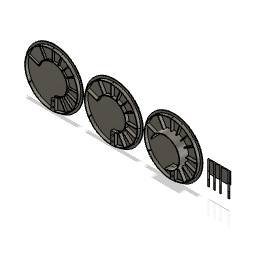
tray2 (Autodesk Fusion 360 design; units mm, degrees)
Autodesk Fusion 360 part; units mm, degrees
sketch "Sketch1" plane through (0, 0, 0) normal (0, 0, 1) x (1, 0, 0)
  circle A0 centre (0, 0) radius 48
  dimension "d1" = 96
  constraint coincident A0.centre origin
  measures "d1" diameter of A0
extrude "Extrude1" add sketch "Sketch1" along normal blind 1 makes body 1
sketch "Sketch2" plane through (0, 0, 1) normal (0, 0, 1) x (1, 0, 0)
  circle A0 centre (0, 0) radius 48
  circle A1 centre (0, 0) radius 44.5
  circle A2 centre (0, 0) radius 24
  line L0 (-21.3923, -12.4423) -> (-37.6324, -21.8186)
  line L1 (-0.3829, -44.4984) -> (-0.2151, -24.9991) construction
  line L2 (0.3829, -44.4984) -> (0.2151, -24.9991) construction
  line L3 (0.5, -43.4971) -> (0.5, -24.9949)
  line L4 (0.3829, -44.4984) -> (0.2151, -24.9991) construction
  line L5 (-0.3829, -44.4984) -> (-0.2151, -24.9991) construction
  line L6 (-0.5, -24.9949) -> (-0.5, -43.4971)
  line L7 (-0.5, -24.9949) -> (-0.5, -43.4971)
  line L8 (0.5, -43.4971) -> (0.5, -24.9949)
  line L9 (18.3655, -16.7159) -> (32.6713, -28.7199)
  line L10 (34.0108, -28.697) -> (18.8273, -16.1775) construction
  line L11 (24.4949, -1) -> (43.4885, -1)
  line L12 (24.4949, -1) -> (43.4885, -1)
  line L13 (33.3229, -27.9613) -> (19.012, -15.953)
  line L14 (33.5176, -29.2715) -> (18.5567, -16.4968) construction
  line L15 (21.1881, 11.801) -> (38.6377, 22.0767) construction
  line L16 (24.9983, -0.2892) -> (24.4991, -0.2935) construction
  line L17 (21.3911, 11.4445) -> (39.0085, 21.4147) construction
  line L18 (37.7117, 21.6814) -> (21.6901, 12.4313)
  line L19 (22.1701, 11.5537) -> (38.2001, 20.8087)
  line L20 (0.5, 23.9949) -> (0.5, 43.4971)
  line L21 (0.5, 23.9949) -> (0.5, 43.4971)
  line L22 (-0.2065, 23.9991) -> (-0.3829, 44.4984) construction
  line L23 (-0.5, 43.4971) -> (-0.5, 23.9949)
  line L24 (-0.5, 43.4971) -> (-0.5, 23.9949)
  line L25 (-0.2065, 23.9991) -> (-0.3829, 44.4984) construction
  line L26 (0.2065, 23.9991) -> (0.3829, 44.4984) construction
  line L27 (0.2065, 23.9991) -> (0.3829, 44.4984) construction
  line L28 (-41.1989, 13.9606) -> (-23.807, 7.6305)
  line L29 (-23.0959, 7.6749) -> (-42.1029, 14.4082) construction
  line L30 (-23.4828, 8.5767) -> (-40.8671, 14.904)
  line L31 (-22.9488, 8.0791) -> (-41.8448, 15.1414) construction
  line L32 (24.9899, -0.7107) -> (24.4991, -0.7065) construction
  line L33 (40.8861, -14.8517) -> (23.5018, -8.5243)
  line L34 (22.8458, -9.3498) -> (40.5339, -15.7877)
  line L35 (43.5, 0) -> (24.4949, 0)
  line L36 (43.5, 0) -> (24.4949, 0)
  line L37 (15.6609, 18.3411) -> (28.8963, 33.8416) construction
  line L38 (16.4495, 18.8259) -> (28.3424, 32.9993)
  line L39 (27.5764, 33.6421) -> (15.6835, 19.4687)
  line L40 (15.3395, 18.6037) -> (28.3097, 34.3338) construction
  line L41 (8.1841, 22.5927) -> (15.0198, 41.8886) construction
  line L42 (14.5672, 40.9884) -> (8.2395, 23.6032)
  line L43 (8.5722, 22.4514) -> (15.7379, 41.6241) construction
  line L44 (9.1769, 23.2548) -> (15.5056, 40.6427)
  line L45 (-12.1471, 21.8506) -> (-21.3978, 37.8733)
  line L46 (-11.9265, 20.9011) -> (-21.9916, 38.6861) construction
  line L47 (-12.3026, 20.6872) -> (-22.6701, 38.2925) construction
  line L48 (-22.2628, 37.3714) -> (-13.0112, 21.3473)
  line L49 (-37.1209, -22.6779) -> (-20.8871, -13.3054)
  line L50 (-38.0463, -23.0809) -> (-21.034, -13.0627) construction
  line L51 (-38.4413, -22.4168) -> (-21.2527, -12.6891) construction
  line L52 (21.8435, -38.77) -> (12.207, -21.7424) construction
  line L53 (11.9505, -21.8877) -> (21.2332, -37.9658)
  line L54 (22.1003, -37.4677) -> (12.8134, -21.3822)
  line L55 (22.4913, -38.3978) -> (12.5611, -21.5349) construction
  line L56 (44.4913, -0.8785) -> (43.4913, -0.8699) construction
  line L57 (24.9899, -0.7107) -> (24.4991, -0.7065) construction
  line L58 (44.4998, -0.1214) -> (43.4998, -0.13) construction
  line L59 (24.9983, -0.2892) -> (24.4991, -0.2935) construction
  line L60 (23.4011, -8.797) -> (23.0915, -8.6873) construction
  line L61 (41.5183, -16.0151) -> (40.5815, -15.665) construction
  line L62 (23.2505, -9.1877) -> (22.9502, -9.0754) construction
  arc A3 (40.8861, -14.8517) -> (43.4913, -0.8699) centre (0, 0) ccw
  arc A4 (19.1511, -16.0697) -> (23.2505, -9.1877) centre (0, 0) ccw
  arc A5 (12.8496, -21.445) -> (18.493, -16.8229) centre (0, 0) ccw
  arc A6 (33.2392, -28.0607) -> (40.5815, -15.665) centre (0, 0) ccw
  arc A7 (21.9839, -37.5361) -> (32.7571, -28.6221) centre (0, 0) ccw
  arc A8 (0.5, -24.995) -> (11.9817, -21.9417) centre (0, 0) ccw
  arc A9 (0.3743, -43.4984) -> (21.3509, -37.8997) centre (0, 0) ccw
  arc A10 (-37.1845, -22.5734) -> (-0.3743, -43.4984) centre (0, 0) ccw
  arc A11 (-21.0908, -13.423) -> (-0.5, -24.995) centre (0, 0) ccw
  arc A12 (-23.7203, 7.8961) -> (-21.6109, -12.5686) centre (0, 0) ccw
  arc A13 (-41.1602, 14.0743) -> (-37.571, -21.9242) centre (0, 0) ccw
  arc A14 (-12.7751, 21.4895) -> (-23.5771, 8.3139) centre (0, 0) ccw
  arc A15 (-22.1626, 37.4308) -> (-40.908, 14.7913) centre (0, 0) ccw
  arc A16 (-0.3743, 43.4984) -> (-21.4991, 37.8158) centre (0, 0) ccw
  arc A17 (14.6859, 40.946) -> (0.3743, 43.4984) centre (0, 0) ccw
  arc A18 (27.6735, 33.5623) -> (15.3878, 40.6874) centre (0, 0) ccw
  arc A19 (8.5082, 23.5077) -> (-12.3873, 21.7153) centre (0, 0) ccw
  arc A20 (15.9043, 19.2887) -> (8.911, 23.358) centre (0, 0) ccw
  arc A21 (21.8321, 12.1803) -> (16.2339, 19.0121) centre (0, 0) ccw
  arc A22 (43.4998, -0.13) -> (38.1381, 20.9221) centre (0, 0) ccw
  arc A23 (37.7759, 21.5692) -> (28.2469, 33.0811) centre (0, 0) ccw
  arc A24 (23.4011, -8.797) -> (24.98, -1) centre (0, 0) ccw
  arc A25 (24.9983, -0.2892) -> (22.0352, 11.8089) centre (0, 0) ccw
  dimension "d4" = 89
  dimension "d5" = 87
  dimension "d6" = 50
  dimension "d7" = 48
  constraint concentric A0 A1
  constraint concentric A0 A22
  constraint concentric A22 A24
  constraint concentric A1 A2
  constraint collinear L0 L18
  constraint collinear L6 L23
  constraint collinear L7 L24
  constraint collinear L28 L34
  constraint coincident A1 L61.start
  constraint coincident A1 L56.start
  constraint coincident A1 L58.start
  constraint coincident A1 L17.end
  constraint coincident A1 L15.end
  constraint coincident A1 L37.end
  constraint coincident A1 L40.end
  constraint coincident A1 L41.end
  constraint coincident A1 L43.end
  constraint coincident A1 L26.end
  constraint coincident A1 L22.end
  constraint coincident A1 L46.end
  constraint coincident A1 L47.end
  constraint coincident A1 L31.end
  constraint coincident A1 L29.end
  constraint coincident A1 L50.start
  constraint coincident A1 L51.start
  constraint coincident A1 L1.start
  constraint coincident A1 L2.start
  constraint coincident A1 L52.start
  constraint coincident A1 L55.start
  constraint coincident A1 L10.start
  constraint coincident A1 L14.start
  constraint coincident L11.end A22
  constraint coincident L35.start A22
  constraint collinear L56 L57
  constraint coincident L16.start A24
  constraint collinear L58 L59
  constraint collinear L61 L62
  constraint coincident L33.start A22
  constraint concentric A3 A22
  constraint coincident L34.end A22
  constraint coincident L33.end A24
  constraint concentric A4 A24
  constraint coincident L13 A4.start
  constraint coincident L9 A5.end
  constraint concentric A5 A24
  constraint coincident L54 A5.start
  constraint coincident L53 A8.end
  constraint coincident L14 A7.end
  constraint coincident L10 A6.start
  constraint concentric A6 A22
  constraint coincident A6 L13.start
  constraint coincident L9.end A22
  constraint coincident L54.start A22
  constraint coincident L53.end A22
  constraint coincident L52 A9.end
  constraint coincident L55 A7.start
  constraint concentric A7 A22
  constraint concentric A8 A24
  constraint coincident L3 A8.start
  constraint coincident L6 A11.end
  constraint coincident L1 A10.end
  constraint coincident L2 A9.start
  constraint concentric A9 A22
  constraint coincident A9 L3.start
  constraint coincident L6.end A22
  constraint coincident L49.start A22
  constraint coincident L0.end A22
  constraint coincident L51 A13.end
  constraint coincident L50 A10.start
  constraint concentric A10 A22
  constraint concentric A11 A24
  constraint coincident L49 A11.start
  constraint coincident L0 A12.end
  constraint coincident L28.end A24
  constraint coincident L30.start A24
  constraint coincident L31 A14.end
  constraint coincident L29 A12.start
  constraint concentric A12 A24
  constraint coincident L31 A15.end
  constraint coincident L29 A13.start
  constraint concentric A13 A22
  constraint coincident A13 L28.start
  constraint coincident L30.end A22
  constraint coincident L46 A19.end
  constraint coincident L47 A14.start
  constraint concentric A14 A24
  constraint coincident A14 L48.end
  constraint coincident L45.start A24
  constraint coincident L46 A16.end
  constraint coincident L47 A15.start
  constraint concentric A15 A22
  constraint coincident L45.end A22
  constraint coincident A15 L48.start
  constraint coincident L26 A17.end
  constraint coincident L22 A16.start
  constraint concentric A16 A22
  constraint coincident L20.end A22
  constraint coincident A16 L23.start
  constraint coincident L44.end A22
  constraint coincident L43 A18.end
  constraint coincident L41 A17.start
  constraint concentric A17 A22
  constraint coincident A17 L42.start
  constraint coincident L37 A23.end
  constraint coincident L40 A18.start
  constraint concentric A18 A22
  constraint coincident L38.end A22
  constraint coincident A18 L39.start
  constraint coincident L43 A20.end
  constraint coincident L41 A19.start
  constraint concentric A19 A24
  constraint coincident L44.start A24
  constraint coincident A19 L42.end
  constraint coincident L39.end A24
  constraint coincident L38.start A24
  constraint coincident L37 A21.end
  constraint coincident L40 A20.start
  constraint concentric A20 A24
  constraint coincident L19.start A24
  constraint coincident L18.end A24
  constraint coincident L17 A25.end
  constraint coincident L15 A21.start
  constraint concentric A21 A24
  constraint coincident L17 A22.end
  constraint coincident L15 A23.start
  constraint concentric A22 A23
  constraint coincident A22 L19.end
  constraint coincident A23 L18.start
  constraint concentric A24 A25
  constraint coincident L11 A24.end
  measures "d4" diameter of A1
  measures "d5" diameter of A22
  measures "d6" diameter of A24
  measures "d7" diameter of A2
extrude "Extrude3" add sketch "Sketch2" along normal blind 5 contours A1 | A2 L20 L21 L23 L24 A19 bodies 1
sketch "Sketch4" plane through (0, 0, 6) normal (0, 0, 1) x (1, 0, 0)
  arc A0 (27.5764, 33.6421) -> (15.5056, 40.6427) centre (0, 0) ccw
  line L0 (27.5764, 33.6421) -> (15.6835, 19.4687)
  arc A1 (15.6835, 19.4687) -> (9.1769, 23.2548) centre (0, 0) ccw
  line L1 (9.1769, 23.2548) -> (15.5056, 40.6427)
  arc A2 (40.8861, -14.8517) -> (43.4885, -1) centre (0, 0) ccw
  line L2 (40.8861, -14.8517) -> (23.5018, -8.5243)
  arc A3 (23.5018, -8.5243) -> (24.98, -1) centre (0, 0) ccw
  line L3 (24.98, -1) -> (43.4885, -1)
  arc A4 (-37.1209, -22.6779) -> (-0.5, -43.4971) centre (0, 0) ccw
  line L4 (-37.1209, -22.6779) -> (-21.0908, -13.423)
  arc A5 (-21.0908, -13.423) -> (-0.5, -24.995) centre (0, 0) ccw
  line L5 (-0.5, -24.995) -> (-0.5, -43.4971)
  arc A6 (0.5, -43.4971) -> (21.2332, -37.9658) centre (0, 0) ccw
  line L6 (0.5, -43.4971) -> (0.5, -24.995)
  arc A7 (0.5, -24.995) -> (11.9817, -21.9417) centre (0, 0) ccw
  line L7 (11.9817, -21.9417) -> (21.2332, -37.9658)
  arc A8 (33.3229, -27.9613) -> (40.5339, -15.7877) centre (0, 0) ccw
  line L8 (33.3229, -27.9613) -> (19.1511, -16.0697)
  arc A9 (19.1511, -16.0697) -> (23.142, -9.4576) centre (0, 0) ccw
  line L9 (23.142, -9.4576) -> (40.5339, -15.7877)
  arc A10 (-0.5, 43.4971) -> (-21.3978, 37.8733) centre (0, 0) ccw
  line L10 (-0.5, 43.4971) -> (-0.5, 24.995)
  arc A11 (-0.5, 24.995) -> (-12.1471, 21.8506) centre (0, 0) ccw
  line L11 (-12.1471, 21.8506) -> (-21.3978, 37.8733)
  arc A12 (14.5672, 40.9884) -> (0.5, 43.4971) centre (0, 0) ccw
  line L12 (14.5672, 40.9884) -> (8.2395, 23.6032)
  arc A13 (8.2395, 23.6032) -> (0.5, 24.995) centre (0, 0) ccw
  line L13 (0.5, 24.995) -> (0.5, 43.4971)
  arc A14 (22.1003, -37.4677) -> (32.6713, -28.7199) centre (0, 0) ccw
  line L14 (22.1003, -37.4677) -> (12.8496, -21.445)
  arc A15 (12.8496, -21.445) -> (18.493, -16.8229) centre (0, 0) ccw
  line L15 (18.493, -16.8229) -> (32.6713, -28.7199)
  arc A16 (37.7117, 21.6814) -> (28.3424, 32.9993) centre (0, 0) ccw
  line L16 (37.7117, 21.6814) -> (21.6901, 12.4313)
  arc A17 (21.6901, 12.4313) -> (16.4495, 18.8259) centre (0, 0) ccw
  line L17 (16.4495, 18.8259) -> (28.3424, 32.9993)
  arc A18 (-22.2628, 37.3714) -> (-40.8671, 14.904) centre (0, 0) ccw
  line L18 (-22.2628, 37.3714) -> (-13.0112, 21.3473)
  arc A19 (-13.0112, 21.3473) -> (-23.4828, 8.5767) centre (0, 0) ccw
  line L19 (-23.4828, 8.5767) -> (-40.8671, 14.904)
  arc A20 (-41.1989, 13.9606) -> (-37.6324, -21.8186) centre (0, 0) ccw
  line L20 (-41.1989, 13.9606) -> (-23.807, 7.6305)
  arc A21 (-23.807, 7.6305) -> (-21.6109, -12.5686) centre (0, 0) ccw
  line L21 (-21.6109, -12.5686) -> (-37.6324, -21.8186)
  arc A22 (43.5, 0) -> (38.2001, 20.8087) centre (0, 0) ccw
  line L22 (43.5, 0) -> (25, 0)
  arc A23 (25, 0) -> (22.1701, 11.5537) centre (0, 0) ccw
  line L23 (22.1701, 11.5537) -> (38.2001, 20.8087)
  circle A24 centre (0, 0) radius 24
  circle A25 centre (0, 0) radius 44.5
  circle A26 centre (0, 0) radius 24
  circle A27 centre (0, 0) radius 25
  constraint concentric A0 A26
  constraint concentric A26 A27
extrude "Extrude4" add sketch "Sketch4" along normal blind 10 contours A1 A3 A5 A7 A9 A11 A13 A15 A17 A19 A21 A23 A27 bodies 1
sketch "Sketch5" plane through (0, 0, 16) normal (0, 0, 1) x (1, 0, 0)
  circle A0 centre (0, 0) radius 24
  circle A1 centre (0, 0) radius 25
  line L0 (-0.5283, -25.9639) -> (-0.7943, 6.8859)
  line L1 (-0.7943, 6.8859) -> (-28.5016, 7.6395)
  line L2 (-28.5016, 7.6395) -> (-37.5896, -21.7967)
  line L3 (-37.5896, -21.7967) -> (-36.969, -22.7277)
  line L4 (-36.969, -22.7277) -> (-0.5283, -25.9639)
extrude "Extrude5" cut sketch "Sketch5" against normal up to surface (15 mm away) contours A0 L0 L1 | A0 A1 L0 L1 | A1 L0 L1 L2 L3 L4 picked at (-1.7694, -13.5925) picked at (-23.4288, 6.3815) bodies 1
sketch "Sketch6" plane through (0, 0, 0) normal (0, 1, 0) x (1, 0, 0)
  line L0 (90, 0) -> (115, -25)
  line L1 (115, -25) -> (116.4142, -23.5858)
  line L2 (92.2226, 0.6058) -> (92.2217, 0.6055)
  line L3 (101, -25) -> (102.4142, -23.5858)
  line L4 (78.2226, 0.6058) -> (78.2217, 0.6055)
  line L5 (76, 0) -> (101, -25)
  line L6 (91, -25) -> (92.4142, -23.5858)
  line L7 (68.2226, 0.6058) -> (68.2217, 0.6055)
  line L8 (66, 0) -> (91, -25)
  line L9 (81, -25) -> (82.4142, -23.5858)
  line L10 (58.2226, 0.6058) -> (58.2217, 0.6055)
  line L11 (56, 0) -> (81, -25)
  line L12 (56, -0.04) -> (56, 0)
  line L13 (92.8684, 0) -> (92.8684, -0.04)
  line L14 (92.8684, -0.04) -> (92.8684, 0.6055)
  line L15 (92.8684, 0.6055) -> (56, 0.6055)
  line L16 (56, 0.6055) -> (56, -0.04)
  line L17 (92.8284, 0) -> (92.8684, 0)
  line L18 (78.8284, 0) -> (90, 0)
  line L19 (102.4142, -23.5858) -> (78.8284, 0)
  line L20 (78.2229, 0.6055) -> (78.2226, 0.6058)
  line L21 (116.4142, -23.5858) -> (92.8284, 0)
  line L22 (92.2229, 0.6055) -> (92.2226, 0.6058)
  line L23 (58.8284, 0) -> (66, 0)
  line L24 (68.8284, 0) -> (76, 0)
  line L25 (56.04, -0.04) -> (56, -0.04)
  line L26 (92.4142, -23.5858) -> (68.8284, 0)
  line L27 (68.2229, 0.6055) -> (68.2226, 0.6058)
  line L28 (56, -0.04) -> (56.04, -0.04)
  line L29 (82.4142, -23.5858) -> (58.8284, 0)
  line L30 (58.2229, 0.6055) -> (58.2226, 0.6058)
  dimension "d29" = 2
  dimension "d30" = 2
  dimension "d31" = 2
  dimension "d32" = 2
  constraint perpendicular L0 L1
  constraint perpendicular L1 L21
  constraint perpendicular L3 L5
  constraint perpendicular L3 L19
  constraint perpendicular L6 L8
  constraint perpendicular L6 L26
  constraint perpendicular L9 L11
  constraint perpendicular L9 L29
  constraint vertical L12
  constraint horizontal L23
  constraint vertical L13
  constraint coincident L13.end L21
  constraint horizontal L28
  constraint vertical L14
  constraint horizontal L15
  constraint vertical L16
  constraint coincident L15 L2.end
  constraint collinear L17 L23
  constraint collinear L18 L23
  constraint coincident L15 L4.end
  constraint coincident L15 L20.start
  constraint collinear L19 L20
  constraint coincident L15 L22.start
  constraint collinear L21 L22
  constraint collinear L23 L24
  constraint coincident L15 L27.start
  constraint collinear L26 L27
  constraint coincident L15 L7.end
  constraint coincident L11 L25.start
  constraint coincident L15 L10.end
  constraint coincident L15 L30.start
  constraint collinear L29 L30
  measures "d29" distance of L0.end L1.end
  measures "d30" distance of L3.end L3.start
  measures "d31" distance of L6.end L6.start
  measures "d32" distance of L9.end L9.start
extrude "Extrude6" add sketch "Sketch6" along normal mid plane 20 separate body contours L0 L1 L3 L5 L6 L8 L9 L11 L14 L15 L16 L17 L18 L19 L21 L23 L24 L26 L29 makes body 2
sketch "Sketch7" plane through (56, 0, 0) normal (-1, 0, 0) x (0, 0, 1)
  line L0 (0, -10) -> (0, 10)
  line L1 (0, 10) -> (-0.6055, 10)
  line L2 (-0.6055, 10) -> (-0.6055, -10)
  line L3 (-0.6055, -10) -> (0, -10)
  line L4 (0, 20) -> (25, 5)
  line L5 (25, 5) -> (25, -5)
  line L6 (25, -5) -> (0, -15)
  line L7 (0, -15) -> (34.4485, -15)
  line L8 (34.4485, -15) -> (34.7895, 20.635)
  line L9 (34.7895, 20.635) -> (0, 20)
  constraint vertical L5
  constraint perpendicular L5 L7
extrude "Extrude7" cut sketch "Sketch7" against normal blind 78 contours L4 L5 L6 L7 L8 L9 bodies 2
extrude "Extrude8" add 1 faces at (80.579, 3.3333, -0.6055) along direction (0, 0, -1) blind 1 on bodies 2 bodies 2
copy_body "CopyPasteBodies1" bodies 1 makes body 3
move_body "Move1" bodies 3 to x (1, 0, 0) y (0, 1, 0) z (0, 0, 1) at (-100, 0, 0)
sketch "Sketch8" plane through (0, 0, 16) normal (0, 0, 1) x (1, 0, 0)
  line L0 (-100.5443, -23.9938) -> (-100.5362, -24.9943)
  arc A0 (-100.5362, -24.9943) -> (-123.8444, 7.5129) centre (-100, 0) ccw
  line L1 (-123.8444, 7.5129) -> (-122.8031, 7.4845)
  arc A1 (-100.5443, -23.9938) -> (-122.8031, 7.4845) centre (-100, 0) ccw
extrude "Extrude9" cut sketch "Sketch8" against normal up to surface (10 mm away) bodies 3
copy_body "CopyPasteBodies2" bodies 1 makes body 4
move_body "Move2" bodies 4 to x (1, 0, 0) y (0, 1, 0) z (0, 0, 1) at (-200, 0, 0)
sketch "Sketch9" plane through (0, 0, 6) normal (0, 0, 1) x (1, 0, 0)
  line L0 (-237.0351, -22.6284) -> (-237.5896, -21.7967)
  line L1 (-237.5896, -21.7967) -> (-237.5885, -21.7932)
  line L2 (-237.5885, -21.7932) -> (-237.6324, -21.8186)
  arc A0 (-241.1989, 13.9606) -> (-237.6324, -21.8186) centre (-200, 0) ccw
  line L3 (-241.1989, 13.9606) -> (-223.807, 7.6305)
  arc A1 (-223.4828, 8.5767) -> (-223.807, 7.6305) centre (-200, 0) ccw
  line L4 (-223.4828, 8.5767) -> (-240.8671, 14.904)
  arc A2 (-222.2628, 37.3714) -> (-240.8671, 14.904) centre (-200, 0) ccw
  line L5 (-222.2628, 37.3714) -> (-213.0112, 21.3473)
  arc A3 (-212.1471, 21.8506) -> (-213.0112, 21.3473) centre (-200, 0) ccw
  line L6 (-212.1471, 21.8506) -> (-221.3978, 37.8733)
  arc A4 (-200.5, 43.4971) -> (-221.3978, 37.8733) centre (-200, 0) ccw
  line L7 (-200.5, 43.4971) -> (-200.5, 24.995)
  arc A5 (-199.5, 24.995) -> (-200.5, 24.995) centre (-200, 0) ccw
  line L8 (-199.5, 24.995) -> (-199.5, 43.4971)
  arc A6 (-185.4328, 40.9884) -> (-199.5, 43.4971) centre (-200, 0) ccw
  line L9 (-185.4328, 40.9884) -> (-191.7605, 23.6032)
  arc A7 (-190.8231, 23.2548) -> (-191.7605, 23.6032) centre (-200, 0) ccw
  line L10 (-190.8231, 23.2548) -> (-184.4944, 40.6427)
  arc A8 (-172.4236, 33.6421) -> (-184.4944, 40.6427) centre (-200, 0) ccw
  line L11 (-172.4236, 33.6421) -> (-184.3165, 19.4687)
  arc A9 (-183.5505, 18.8259) -> (-184.3165, 19.4687) centre (-200, 0) ccw
  line L12 (-183.5505, 18.8259) -> (-171.6576, 32.9993)
  arc A10 (-162.2883, 21.6814) -> (-171.6576, 32.9993) centre (-200, 0) ccw
  line L13 (-162.2883, 21.6814) -> (-178.3099, 12.4313)
  arc A11 (-177.8299, 11.5537) -> (-178.3099, 12.4313) centre (-200, 0) ccw
  line L14 (-177.8299, 11.5537) -> (-161.7999, 20.8087)
  arc A12 (-156.5, 0) -> (-161.7999, 20.8087) centre (-200, 0) ccw
  line L15 (-156.5, 0) -> (-175, 0)
  arc A13 (-175.02, -1) -> (-175, 0) centre (-200, 0) ccw
  line L16 (-175.02, -1) -> (-156.5115, -1)
  arc A14 (-159.1139, -14.8517) -> (-156.5115, -1) centre (-200, 0) ccw
  line L17 (-159.1139, -14.8517) -> (-176.4982, -8.5243)
  arc A15 (-176.858, -9.4576) -> (-176.4982, -8.5243) centre (-200, 0) ccw
  line L18 (-176.858, -9.4576) -> (-159.4661, -15.7877)
  arc A16 (-166.6771, -27.9613) -> (-159.4661, -15.7877) centre (-200, 0) ccw
  line L19 (-166.6771, -27.9613) -> (-180.8489, -16.0697)
  arc A17 (-181.507, -16.8229) -> (-180.8489, -16.0697) centre (-200, 0) ccw
  line L20 (-181.507, -16.8229) -> (-167.3287, -28.7199)
  arc A18 (-177.8997, -37.4677) -> (-167.3287, -28.7199) centre (-200, 0) ccw
  line L21 (-177.8997, -37.4677) -> (-187.1504, -21.445)
  arc A19 (-188.0183, -21.9417) -> (-187.1504, -21.445) centre (-200, 0) ccw
  line L22 (-188.0183, -21.9417) -> (-178.7668, -37.9658)
  arc A20 (-199.5, -43.4971) -> (-178.7668, -37.9658) centre (-200, 0) ccw
  line L23 (-199.5, -43.4971) -> (-199.5, -24.995)
  arc A21 (-200.5, -24.995) -> (-199.5, -24.995) centre (-200, 0) ccw
  line L24 (-200.5, -24.995) -> (-200.5, -43.4971)
  arc A22 (-237.1209, -22.6779) -> (-200.5, -43.4971) centre (-200, 0) ccw
  line L25 (-237.1209, -22.6779) -> (-237.0351, -22.6284)
  circle A23 centre (-200, 0) radius 44.5
  circle A24 centre (-200, 0) radius 43.5
  constraint concentric A0 A24
extrude "Extrude10" cut sketch "Sketch9" along normal blind 53 and the other way blind 2 contours L0 L1 L2 A0 L3 A1 L4 A2 L5 A3 L6 A4 L7 A5 L8 A6 L9 A7 L10 A8 L11 A9 L12 A10 L13 A11 L14 A12 L15 A13 L16 A14 L17 A15 L18 A16 L19 A17 L20 A18 L21 A19 L22 A20 L23 A21 L24 A22 L25 A24 | L23 A21 L24 A24 | L3 A1 L4 A24 | L21 A19 L22 A24 | L5 A3 L6 A24 | L19 A17 L20 A24 | L7 A5 L8 A24 | L17 A15 L18 A24 | L9 A7 L10 A24 | L15 A13 L16 A24 | L11 A9 L12 A24 | L13 A11 L14 A24 bodies 4
sketch "Sketch10" plane through (0, 0, 1) normal (0, 0, 1) x (1, 0, 0)
  line L0 (21.2332, -37.9658) -> (11.9817, -21.9417)
  arc A0 (0.5, -24.995) -> (11.9817, -21.9417) centre (0, 0) ccw
  line L1 (0.5, -24.995) -> (0.5, -43.4971)
  arc A1 (0.5, -43.4971) -> (21.2332, -37.9658) centre (0, 0) ccw
  line L2 (0, -44) -> (0, -24.51)
  line L3 (0, -24.51) -> (5.9938, -23.7435)
  line L4 (5.9938, -23.7435) -> (5.9938, -43.6025)
  line L5 (5.9938, -43.6025) -> (0, -44)
  circle A2 centre (3, -38) radius 1.2243
  circle A3 centre (3, -29) radius 1.2584
  constraint vertical L2
  constraint parallel L2 L4
extrude "Extrude11" add sketch "Sketch10" along normal blind 5 separate body contours A0 L1 A1 L2 L3 L4 L5 | A0 L1 A1 L4 makes body 5
copy_body "CopyPasteBodies3" bodies 5 makes body 6
move_body "Move3" bodies 6 to x (1, 0, 0) y (0, 1, 0) z (0, 0, 1) at (-100, 0, 0)
copy_body "CopyPasteBodies4" bodies 5 makes body 7
move_body "Move4" bodies 7 to x (1, 0, 0) y (0, 1, 0) z (0, 0, 1) at (-200, 0, 0)
sketch "Sketch11" plane through (0, 0, 4) normal (0, 0, 1) x (1, 0, 0)
  line L0 (-159.1139, -14.8517) -> (-176.4982, -8.5243)
  arc A0 (-176.4982, -8.5243) -> (-175.02, -1) centre (-200, 0) ccw
  line L1 (-175.02, -1) -> (-156.5115, -1)
  arc A1 (-156.5115, -1) -> (-156.5, 0) centre (-200, 0) ccw
  line L2 (-156.5, 0) -> (-175, 0)
  arc A2 (-175, 0) -> (-177.8299, 11.5537) centre (-200, 0) ccw
  line L3 (-177.8299, 11.5537) -> (-161.7999, 20.8087)
  arc A3 (-161.7999, 20.8087) -> (-162.2883, 21.6814) centre (-200, 0) ccw
  line L4 (-162.2883, 21.6814) -> (-178.3099, 12.4313)
  arc A4 (-178.3099, 12.4313) -> (-183.5505, 18.8259) centre (-200, 0) ccw
  line L5 (-183.5505, 18.8259) -> (-171.6576, 32.9993)
  arc A5 (-171.6576, 32.9993) -> (-172.4236, 33.6421) centre (-200, 0) ccw
  line L6 (-172.4236, 33.6421) -> (-184.3165, 19.4687)
  arc A6 (-184.3165, 19.4687) -> (-190.8231, 23.2548) centre (-200, 0) ccw
  line L7 (-190.8231, 23.2548) -> (-184.4944, 40.6427)
  arc A7 (-184.4944, 40.6427) -> (-185.4328, 40.9884) centre (-200, 0) ccw
  line L8 (-185.4328, 40.9884) -> (-191.7605, 23.6032)
  arc A8 (-191.7605, 23.6032) -> (-199.5, 24.995) centre (-200, 0) ccw
  line L9 (-199.5, 24.995) -> (-199.5, 43.4971)
  arc A9 (-199.5, 43.4971) -> (-200.5, 43.4971) centre (-200, 0) ccw
  line L10 (-200.5, 43.4971) -> (-200.5, 24.995)
  arc A10 (-200.5, 24.995) -> (-212.1471, 21.8506) centre (-200, 0) ccw
  line L11 (-212.1471, 21.8506) -> (-221.3978, 37.8733)
  arc A11 (-221.3978, 37.8733) -> (-222.2628, 37.3714) centre (-200, 0) ccw
  line L12 (-222.2628, 37.3714) -> (-213.0112, 21.3473)
  arc A12 (-213.0112, 21.3473) -> (-223.4828, 8.5767) centre (-200, 0) ccw
  line L13 (-223.4828, 8.5767) -> (-240.8671, 14.904)
  arc A13 (-240.8671, 14.904) -> (-241.1989, 13.9606) centre (-200, 0) ccw
  line L14 (-241.1989, 13.9606) -> (-223.807, 7.6305)
  arc A14 (-223.807, 7.6305) -> (-223.8444, 7.5129) centre (-200, 0) ccw
  line L15 (-223.8444, 7.5129) -> (-222.8031, 7.4845)
  arc A15 (-200.5443, -23.9938) -> (-222.8031, 7.4845) centre (-200, 0) ccw
  line L16 (-200.5443, -23.9938) -> (-200.5362, -24.9942)
  arc A16 (-200.5362, -24.9942) -> (-200.5, -24.995) centre (-200, 0) ccw
  line L17 (-200.5, -24.995) -> (-200.5, -43.4971)
  arc A17 (-200.5, -43.4971) -> (-199.5, -43.4971) centre (-200, 0) ccw
  line L18 (-199.5, -43.4971) -> (-199.5, -24.995)
  arc A18 (-199.5, -24.995) -> (-188.0183, -21.9417) centre (-200, 0) ccw
  line L19 (-188.0183, -21.9417) -> (-178.7668, -37.9658)
  arc A19 (-178.7668, -37.9658) -> (-177.8997, -37.4677) centre (-200, 0) ccw
  line L20 (-177.8997, -37.4677) -> (-187.1504, -21.445)
  arc A20 (-187.1504, -21.445) -> (-181.507, -16.8229) centre (-200, 0) ccw
  line L21 (-181.507, -16.8229) -> (-167.3287, -28.7199)
  arc A21 (-167.3287, -28.7199) -> (-166.6771, -27.9613) centre (-200, 0) ccw
  line L22 (-166.6771, -27.9613) -> (-180.8489, -16.0697)
  arc A22 (-180.8489, -16.0697) -> (-176.858, -9.4576) centre (-200, 0) ccw
  line L23 (-176.858, -9.4576) -> (-159.4661, -15.7877)
  arc A23 (-159.4661, -15.7877) -> (-159.1139, -14.8517) centre (-200, 0) ccw
  line L24 (-194, -25) -> (-194, -23.2379)
  constraint coincident A15 L24.end
  constraint vertical L24
extrude "Extrude12" add sketch "Sketch11" along normal up to surface (2 mm away) contours A15 L16 A16 L17 A17 L18 A18 L24 bodies 4 7
sketch "Sketch12" plane through (0, 0, 6) normal (0, 0, 1) x (1, 0, 0)
  arc A0 (-237.1209, -22.6779) -> (-200.5, -43.4971) centre (-200, 0) ccw
  line L0 (-237.1209, -22.6779) -> (-237.0351, -22.6284)
  line L1 (-237.0351, -22.6284) -> (-237.5896, -21.7967)
  line L2 (-237.5896, -21.7967) -> (-237.5885, -21.7932)
  line L3 (-237.5885, -21.7932) -> (-237.6324, -21.8186)
  arc A1 (-194.0062, -43.0851) -> (-237.6324, -21.8186) centre (-200, 0) ccw
  line L4 (-194.0062, -43.0851) -> (-194.0062, -24.2709)
  arc A2 (-194.0062, -24.2709) -> (-194, -24.2693) centre (-200, 0) ccw
  line L5 (-194, -24.2693) -> (-194, -23.2379)
  arc A3 (-200.5443, -23.9938) -> (-194, -23.2379) centre (-200, 0) ccw
  line L6 (-200.5443, -23.9938) -> (-200.5362, -24.9942)
  arc A4 (-200.5362, -24.9942) -> (-200.5, -24.995) centre (-200, 0) ccw
  line L7 (-200.5, -24.995) -> (-200.5, -43.4971)
  circle A5 centre (-197, -29) radius 1.2584
  circle A6 centre (-197, -38) radius 1.2243
  circle A7 centre (-200, 0) radius 44.5
  line L8 (-200.5, -43.4971) -> (-200, -23)
  line L9 (-200, -23) -> (-203.5921, -23.9938)
  line L10 (-203.5921, -23.9938) -> (-200.5, -43.4971)
  constraint coincident A0.end L7.end
extrude "Extrude13" cut sketch "Sketch12" against normal up to surface (5 mm away) contours A3 L6 A4 L7 L8 L9 L10 | A3 L6 A4 L7 L8 bodies 4
fillet "Fillet1" radius 5 1 edges at (-200.0244, -24, 3.5) on bodies 4
combine "Combine1" operation add target body 5 tool bodies 1
combine "Combine2" operation add target body 3 tool bodies 6
named bodies: "tray2-1", "tilted-support", "tray2-2", "tray2-3", "balance-support", "balance-support (1)", "balance-support (1) (1)"
